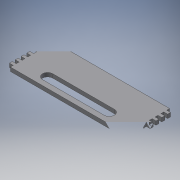
# Autodesk Inventor part: cabinet-bottom
Saved by Autodesk Inventor 2016 (Build 200138000, 138)
## iProperties
Created: 2015-10-24
Part Number: cabinet-bottom
Material: Wood (Birch)
Document SubType Name: Modeling
Designer: jeremyhale
Density: 0.55 g/cm^3
Appearance: Birch - Natural Polished
Mass: 1187.42 g
Surface Area: 2767.06 cm^2
Volume: 2158.95 cm^3
Author: jeremyhale
Autodesk Inventor part; units mm, degrees
ref_plane "YZ Plane" through (0, 0, 0) normal (1, 0, 0) x (0, 1, 0)
ref_plane "XZ Plane" through (0, 0, 0) normal (0, 1, 0) x (-1, 0, 0)
ref_plane "XY Plane" through (0, 0, 0) normal (0, 0, 1) x (1, 0, 0)
sketch "Sketch1" plane through (0, 0, 0) normal (0, 1, 0) x (-1, 0, 0)
  line L0 (304.8, 107.95) -> (-304.8, 107.95)
  line L1 (-304.8, 107.95) -> (-304.8, -107.95)
  line L2 (-304.8, -107.95) -> (304.8, -107.95)
  line L3 (304.8, -107.95) -> (304.8, 107.95)
  line L4 (304.8, 107.95) -> (-304.8, -107.95) construction
  line L5 (-304.8, 107.95) -> (304.8, -107.95) construction
  point P0 (0, 0)
  dimension "length" = 609.6
  dimension "width" = 215.9
  constraints: 12 end point, 2 midpoint, 2 parallel, 1 horizontal, 1 perpendicular
  measures "length" distance of L2.end L1.end
  measures "width" distance of L1.end L0.end
extrude "Extrusion1" add sketch "Sketch1" along normal blind 19
sketch "Sketch3" plane through (0, 19, 0) normal (0, 1, 0) x (1, 0, 0)
  line L0 (-304.8, 107.95) -> (-304.8, -107.95) projected
  line L1 (-304.8, -107.95) -> (304.8, -107.95) projected
  line L2 (-304.8, -107.95) -> (-285.8, -107.95)
  line L3 (-285.8, -107.95) -> (-285.8, -93.5567)
  line L4 (-285.8, -93.5567) -> (-304.8, -93.5567)
  line L5 (-304.8, -93.5567) -> (-304.8, -107.95)
  point P0 (0, 0)
  dimension "d21" = 19
  dimension "d22" = 14.3933
  constraints: 8 end point, 2 parallel, 1 horizontal, 1 perpendicular
  measures "d21" distance of L4.end L3.end
  measures "d22" distance of L3.end L2.end
extrude "Extrusion3" cut sketch "Sketch3" against normal through all
mirror "Mirror2" about plane through (0, 0, 0) normal (0, 0, 1) of "Extrusion3"
sketch "Sketch4" plane through (0, 19, 0) normal (0, 1, 0) x (1, 0, 0)
  line L0 (-304.8, 93.5567) -> (-304.8, -93.5567) projected
  line L1 (-304.8, -79.1633) -> (-285.8, -79.1633)
  line L2 (-285.8, -79.1633) -> (-285.8, -64.77)
  line L3 (-285.8, -64.77) -> (-304.8, -64.77)
  line L4 (-304.8, -64.77) -> (-304.8, -79.1633)
  line L5 (-304.8, -93.5567) -> (-285.8, -93.5567) projected
  point P0 (0, 0)
  dimension "d25" = 19
  dimension "d26" = 14.3933
  dimension "d27" = 14.3933
  constraints: 8 end point, 2 parallel, 1 horizontal, 1 perpendicular, 1 point on line
  measures "d25" distance of L3.end L2.end
  measures "d26" distance of L2.end L1.end
  measures "d27" distance between parallel lines of L5 L1
extrude "Extrusion4" cut sketch "Sketch4" against normal through all
pattern_linear "Rectangular Pattern1" count 6 spacing 28.7867 along (0, 0, -1) of "Extrusion4"
mirror "Mirror3" about plane through (0, 0, 0) normal (1, 0, 0) of "Extrusion3", "Mirror2", "Extrusion4", "Rectangular Pattern1"
sketch "Sketch5" plane through (0, 0, 0) normal (0, -1, 0) x (1, 0, 0)
  circle A0 centre (-108.425, 56.675) radius 15 construction
  circle A1 centre (-44.925, 56.675) radius 15 construction
  circle A2 centre (18.575, 56.675) radius 15 construction
  circle A3 centre (82.075, 56.675) radius 15 construction
  circle A4 centre (145.575, 56.675) radius 15 construction
  circle A5 centre (209.075, 56.675) radius 15 construction
  line L0 (152.4, 57.15) -> (-152.4, 57.15) construction
  line L1 (152.4, 76.2) -> (-152.4, 76.2)
  line L2 (-152.4, 38.1) -> (152.4, 38.1)
  arc A6 (152.4, 38.1) -> (152.4, 76.2) centre (152.4, 57.15) ccw
  arc A7 (-152.4, 76.2) -> (-152.4, 38.1) centre (-152.4, 57.15) ccw
  line L3 (-285.8, 107.95) -> (285.8, 107.95) projected
  point P0 (0, 0)
  point P1 (0, 57.15)
  dimension "d33" = 38.1
  dimension "d34" = 304.8
  dimension "d35" = 0
  dimension "d36" = 50.8
  constraints: 8 end point, 4 point on circle, 4 tangent, 2 centre point, 1 horizontal, 1 midpoint, 1 parallel
  measures "d33" diameter of A7
  measures "d34" distance of L0.end L0.start
  measures "d35" horizontal distance of point (0, 0) point (0, 57.15)
  measures "d36" distance from line of L3 L0.end
extrude "Extrusion5" cut sketch "Sketch5" against normal blind 19
chamfer "Chamfer1" distance 3.175 angle 45 20 edges at (-171.45, 0, 57.15) (0, 0, 76.2) (171.45, 0, 57.15) (0, 0, 38.1) (0, 0, -107.95) (0, 0, 107.95) (304.8, 0, 86.36) (304.8, 0, 57.5733) (304.8, 0, 28.7867) (304.8, 0, 0) (304.8, 0, -28.7867) (304.8, 0, -57.5733) (304.8, 0, -86.36) (-304.8, 0, 86.36) (-304.8, 0, 57.5733) (-304.8, 0, 28.7867) (-304.8, 0, 0) (-304.8, 0, -28.7867) (-304.8, 0, -57.5733) (-304.8, 0, -86.36)
chamfer "Chamfer2" distance 3.175 angle 45 2 edges at (0, 19, -107.95) (0, 19, 107.95)
equation "\"d21\" = thickness"
equation "\"d25\" = thickness"
equation "\"d37\" = thickness"
equation "\"thickness\" = 19"
body "Solid1"
